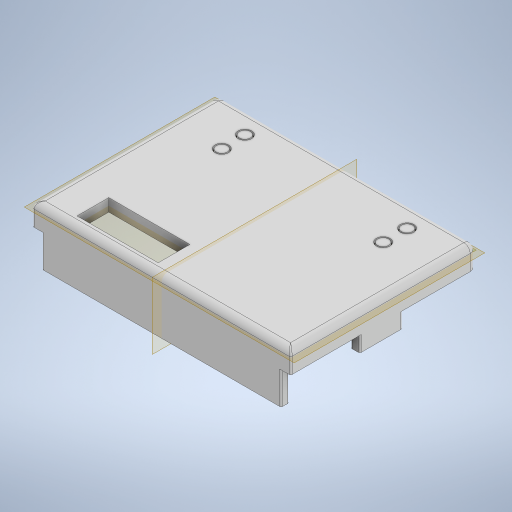
# Autodesk Inventor part: dach
Saved by Autodesk Inventor 2023 (Build 270158000, 158)
## iProperties
Created: 2024-04-28
Part Number: dach
Material: Ogólny
Document SubType Name: Modeling
Designer: kamil
Density: 1 g/cm^3
Appearance: Domyślna
Author: kamil
Autodesk Inventor part; units mm, degrees
ref_plane "YZ Plane" through (0, 0, 0) normal (1, 0, 0) x (0, 1, 0)
ref_plane "XZ Plane" through (0, 0, 0) normal (0, 1, 0) x (-1, 0, 0)
ref_plane "XY Plane" through (0, 0, 0) normal (0, 0, 1) x (1, 0, 0)
sketch "Szkic1" plane through (0, 0, 0) normal (0, 1, 0) x (-1, 0, 0)
  line L0 (41, 29.5365) -> (-41, 29.5365)
  line L1 (-41, 29.5365) -> (-41, -29.5365)
  line L2 (-41, -29.5365) -> (41, -29.5365)
  line L3 (41, -29.5365) -> (41, 29.5365)
  point P0 (0, 0)
  point P1 (41, 0)
  point P2 (0, -29.5365)
  dimension "d0" = 82
  dimension "d1" = 59.073
  constraints: 8 end point, 2 midpoint, 2 parallel, 1 horizontal, 1 horizontal alignment, 1 perpendicular, 1 vertical alignment
  measures "d0" distance of L1.end L2.end
  measures "d1" distance of L2.end L0.start
extrude "Wyciągnięcie proste1" add sketch "Szkic1" along normal blind 4
fillet "Zaokrąglenie2" radius 2 2 edges at (41, 2, -29.5365) (-41, 2, -29.5365)
sketch "Szkic3" plane through (0, 0, 0) normal (0, -1, 0) x (1, 0, 0)
  line L0 (41, 29.5365) -> (41, -29.5365) projected
  line L1 (-41, 29.5365) -> (41, 29.5365) projected
  line L2 (-41, -29.5365) -> (-41, 29.5365) projected
  line L3 (38, 27.0365) -> (-38, 27.0365)
  line L4 (-38, 27.0365) -> (-38, 29.5365)
  line L5 (-38, 29.5365) -> (38, 29.5365)
  line L6 (38, 29.5365) -> (38, 27.0365)
  point P0 (0, 0)
  point P1 (41, 15.9365)
  point P2 (-41, 15.9365)
  point P3 (0, 27.0365)
  point P4 (0, 29.5365)
  point P5 (0, 29.5365)
  point P6 (0, 29.5365)
  dimension "d24" = 76
  dimension "d25" = 2.5
  constraints: 8 end point, 4 midpoint, 2 parallel, 1 coincident, 1 horizontal, 1 perpendicular, 1 vertical alignment
  measures "d24" distance of L4.end L5.end
  measures "d25" distance of L3.end L4.end
extrude "Wyciągnięcie proste3" add sketch "Szkic3" along normal blind 13.3
fillet "Zaokrąglenie5" radius 0.5 2 edges at (-41, 2, 29.5365) (41, 2, 29.5365)
fillet "Zaokrąglenie7" radius 2 8 edges at (40.4142, 4, -28.9507) (0, 4, -29.5365) (-40.4142, 4, -28.9507) (-41, 4, 0.75) (-40.8536, 4, 29.3901) (0, 4, 29.5365) (40.8536, 4, 29.3901) (41, 4, 0.75)
ref_plane "Płaszczyzna konstrukcyjna1" through (0, 1.75, 0) normal (0, 1, 0) x (1, 0, 0)
sketch "Szkic6" plane through (0, 0, 0) normal (0, -1, 0) x (1, 0, 0)
  arc A0 (41, 29.0365) -> (40.5, 29.5365) centre (40.5, 29.0365) ccw projected
  line L0 (38, 29.5365) -> (40.5, 29.5365) projected
  line L1 (38, 29.5365) -> (38, 27.0365) projected
  line L2 (38, 27.0365) -> (-38, 27.0365) projected
  line L3 (-38, 27.0365) -> (-38, 29.5365) projected
  line L4 (-40.5, 29.5365) -> (-38, 29.5365) projected
  arc A1 (-40.5, 29.5365) -> (-41, 29.0365) centre (-40.5, 29.0365) ccw projected
  line L5 (-41, -27.5365) -> (-41, 29.0365) projected
  arc A2 (-41, -27.5365) -> (-39, -29.5365) centre (-39, -27.5365) ccw projected
  line L6 (39, -29.5365) -> (-39, -29.5365) projected
  arc A3 (39, -29.5365) -> (41, -27.5365) centre (39, -27.5365) ccw projected
  line L7 (41, 29.0365) -> (41, -27.5365) projected
  line L8 (-38.1, 24.1365) -> (38.1, 24.1365)
  line L9 (38.1, 24.1365) -> (38.1, -26.6365)
  line L10 (38.1, -26.6365) -> (-38.1, -26.6365)
  line L11 (-38.1, -26.6365) -> (-38.1, 24.1365)
  line L12 (-38.1, 24.1365) -> (-38.1, 32.3252)
  line L13 (38.1, 24.1365) -> (38.1, 40.7001)
  line L14 (38.1, 29.5365) -> (-38.1, 29.5365)
  line L15 (-38.1, 29.5365) -> (-38.1, 27.0365)
  line L16 (-38.1, 27.0365) -> (38.1, 27.0365)
  line L17 (38.1, 27.0365) -> (38.1, 29.5365)
  point P0 (0, 0)
  dimension "d71" = 2.9
  constraints: 20 end point, 3 point on line, 2 parallel, 2 vertical, 1 horizontal, 1 perpendicular, 3 other
  measures "d71" distance between parallel lines of L5 L11
extrude "Wyciągnięcie proste4" add sketch "Szkic6" along normal blind 3 contours L7 A3 L6 A2 L5 A1 L4 L12 L11 L10 L9 L13 L0 A0 | L13 L16 L1 L0 | L1 L2 L3 L14 | L3 L16 L12 L4
sketch "Szkic7" plane through (0, 0, 0) normal (0, -1, 0) x (1, 0, 0)
  circle A0 centre (36.5, 0.75) radius 2 projected
  arc A1 (32, -1.25) -> (36.3571, -6.2085) centre (37, -1.25) ccw projected
  line L0 (32, -1.25) -> (32, 2.75) projected
  arc A2 (36.3571, 7.7085) -> (32, 2.75) centre (37, 2.75) ccw projected
  arc A3 (36.3571, 7.7085) -> (38.1, 9.6919) centre (36.1, 9.6919) ccw projected
  line L1 (38.1, 8.25) -> (38.1, 9.6919) projected
  arc A4 (38.1, 8.25) -> (38.6, 7.75) centre (38.6, 8.25) ccw projected
  line L2 (38.6, 7.75) -> (40.5, 7.75) projected
  arc A5 (40.5, 7.75) -> (41, 8.25) centre (40.5, 8.25) ccw projected
  line L3 (41, 8.25) -> (41, -6.75) projected
  arc A6 (41, -6.75) -> (40.5, -6.25) centre (40.5, -6.75) ccw projected
  line L4 (40.5, -6.25) -> (38.6, -6.25) projected
  arc A7 (38.6, -6.25) -> (38.1, -6.75) centre (38.6, -6.75) ccw projected
  line L5 (38.1, -8.1919) -> (38.1, -6.75) projected
  arc A8 (38.1, -8.1919) -> (36.3571, -6.2085) centre (36.1, -8.1919) ccw projected
  circle A9 centre (36.5, 0.75) radius 1.6 projected
  point P0 (0, 0)
extrude "Wyciągnięcie proste5" add sketch "Szkic7" along normal up to surface (3 mm away) contours A0 | L0 A2 A3 L1 A4 L2 A5 L3 A6 L4 A7 L5 A8 A1
sketch "Szkic8" plane through (0, -3, 0) normal (0, -1, 0) x (1, 0, 0)
  line L0 (38.6, -6.25) -> (40.5, -6.25) projected
  line L1 (40.5, 7.75) -> (38.6, 7.75) projected
  circle A0 centre (36.5, 0.75) radius 2 projected
  arc A1 (32, -1.25) -> (36.3571, -6.2085) centre (37, -1.25) ccw projected
  line L2 (32, -1.25) -> (32, 2.75) projected
  arc A2 (36.3571, 7.7085) -> (32, 2.75) centre (37, 2.75) ccw projected
  arc A3 (36.3571, 7.7085) -> (38.1, 9.6919) centre (36.1, 9.6919) ccw projected
  line L3 (38.1, 8.25) -> (38.1, 9.6919) projected
  arc A4 (38.1, 8.25) -> (38.6, 7.75) centre (38.6, 8.25) ccw projected
  line L4 (38.6, 7.75) -> (40.5, 7.75) projected
  arc A5 (40.5, 7.75) -> (41, 8.25) centre (40.5, 8.25) ccw projected
  line L5 (41, 8.25) -> (41, -6.75) projected
  arc A6 (41, -6.75) -> (40.5, -6.25) centre (40.5, -6.75) ccw projected
  line L6 (40.5, -6.25) -> (38.6, -6.25) projected
  arc A7 (38.6, -6.25) -> (38.1, -6.75) centre (38.6, -6.75) ccw projected
  line L7 (38.1, -8.1919) -> (38.1, -6.75) projected
  arc A8 (38.1, -8.1919) -> (36.3571, -6.2085) centre (36.1, -8.1919) ccw projected
  line L8 (41, -6.05) -> (38.1, -6.05)
  line L9 (38.1, -6.05) -> (38.1, 7.55)
  line L10 (38.1, 7.55) -> (41, 7.55)
  line L11 (41, 7.55) -> (41, -6.05)
  point P0 (0, 0)
  point P1 (41, 0.75)
  point P2 (38.1, 0.75)
  dimension "d76" = 0.2
  dimension "d77" = 0.2
  constraints: 8 end point, 2 midpoint, 2 parallel, 2 vertical alignment, 1 horizontal, 1 perpendicular
  measures "d76" distance between parallel lines of L0 L8
  measures "d77" distance between parallel lines of L1 L10
extrude "Wyciągnięcie proste6" add sketch "Szkic8" along normal blind 4.9 contours L8 L9 A0 L10 L5 | L9 A0 picked at (38.2333, 0.75)
fillet "Zaokrąglenie12" radius 0.5 4 edges at (41, -5.45, 7.55) (38.1, -5.45, 7.55) (41, -5.45, -6.05) (38.1, -5.45, -6.05)
ref_plane "Płaszczyzna konstrukcyjna2" through (0, 2, 29.0365) normal (1, 0, 0) x (0, 0, -1)
mirror "Odbij1" about plane through (0, 2, 29.0365) normal (1, 0, 0) of "Zaokrąglenie12", "Wyciągnięcie proste6", "Wyciągnięcie proste5"
fillet "Zaokrąglenie13" radius 0.5 4 edges at (38, -8.15, 29.5365) (38, -8.15, 27.0365) (-38, -8.15, 27.0365) (-38, -8.15, 29.5365)
fillet "Zaokrąglenie14" radius 1 4 edges at (-38.1, -1.5, 27.0365) (38.1, -1.5, 27.0365) (38.1, -1.5, -26.6365) (-38.1, -1.5, -26.6365)
sketch "Szkic9" plane through (0, 4, 0) normal (0, 1, 0) x (1, 0, 0)
  circle A0 centre (-25.3, 14.8865) radius 1.65 projected
  circle A1 centre (-25.5, 22.4365) radius 1.65 projected
  circle A2 centre (26.05, 14.8365) radius 1.65 projected
  circle A3 centre (26.05, 22.4365) radius 1.65 projected
  line L0 (-28.825, -17.5035) -> (-28.825, -25.6035) projected
  line L1 (-28.825, -25.6035) -> (-8.525, -25.6035) projected
  line L2 (-28.825, -17.5035) -> (-8.525, -17.5035)
  line L3 (-8.525, -17.5035) -> (-8.525, -25.6035)
  line L4 (-8.525, -25.6035) -> (-28.825, -25.6035)
  line L5 (-28.825, -25.6035) -> (-28.825, -17.5035)
  point P0 (0, 0)
  constraints: 8 end point, 2 parallel, 1 horizontal, 1 perpendicular
extrude "Wyciągnięcie proste7" cut sketch "Szkic9" against normal blind 5
sketch "Szkic10" plane through (0, 0, 0) normal (0, -1, 0) x (1, 0, 0)
  circle A0 centre (-25.3, -14.8865) radius 1.65 projected
  circle A1 centre (-25.5, -22.4365) radius 1.65 projected
  circle A2 centre (26.05, -22.4365) radius 1.65 projected
  circle A3 centre (26.05, -14.8365) radius 1.65 projected
  circle A4 centre (-25.5, -22.4365) radius 2.15
  circle A5 centre (-25.3, -14.8865) radius 2.15
  circle A6 centre (26.05, -22.4365) radius 2.15
  circle A7 centre (26.05, -14.8365) radius 2.15
  point P0 (0, 0)
  dimension "d86" = 0.5
  dimension "d87" = 0.5
  dimension "d88" = 0.5
  dimension "d89" = 0.5
  constraints: 4 centre point
  measures "d86" radial gap between concentric circles of A1 A4
  measures "d87" radial gap between concentric circles of A0 A5
  measures "d88" radial gap between concentric circles of A2 A6
  measures "d89" radial gap between concentric circles of A3 A7
extrude "Wyciągnięcie proste8" cut sketch "Szkic10" against normal through all contours A0 | A1 | A2 | A3 | A4 | A5 | A6 | A7
sketch "Szkic11" plane through (0, 4, 0) normal (0, 1, 0) x (1, 0, 0)
  circle A0 centre (-25.5, 22.4365) radius 2.15 projected
  circle A1 centre (-25.3, 14.8865) radius 2.15 projected
  circle A2 centre (26.05, 22.4365) radius 2.15 projected
  circle A3 centre (26.05, 14.8365) radius 2.15 projected
  circle A4 centre (-25.5, 22.4365) radius 1.75
  circle A5 centre (-25.3, 14.8865) radius 1.75
  circle A6 centre (26.05, 22.4365) radius 1.75
  circle A7 centre (26.05, 14.8365) radius 1.75
  point P0 (0, 0)
  dimension "d92" = 3.5
  dimension "d93" = 3.5
  dimension "d94" = 3.5
  dimension "d95" = 3.5
  constraints: 4 centre point, 4 coincident
  measures "d92" diameter of A4
  measures "d93" diameter of A5
  measures "d94" diameter of A6
  measures "d95" diameter of A7
extrude "Wyciągnięcie proste9" add sketch "Szkic11" against normal blind 5 contours A4 | A5 | A6 | A7
ref_plane "Płaszczyzna konstrukcyjna3" through (26.05, -2, -22.4365) normal (0, -1, 0) x (1, 0, 0)
sketch "Szkic14" plane through (0, 0, 0) normal (0, -1, 0) x (1, 0, 0)
  circle A0 centre (26.05, -22.4365) radius 2.15 projected
  circle A1 centre (-25.3, -14.8865) radius 2.15 projected
  circle A2 centre (26.05, -14.8365) radius 2.15 projected
  circle A3 centre (-25.5, -22.4365) radius 2.15 projected
  line L0 (-28.825, 17.5035) -> (-28.825, 25.6035) projected
  line L1 (-28.825, 25.6035) -> (-8.525, 25.6035) projected
  line L2 (-8.525, 25.6035) -> (-8.525, 17.5035) projected
  line L3 (-8.525, 17.5035) -> (-28.825, 17.5035) projected
  circle A4 centre (26.05, -22.4365) radius 3.2
  circle A5 centre (26.05, -14.8365) radius 3.2
  circle A6 centre (-25.5, -22.4365) radius 1.75 projected
  circle A7 centre (-25.5, -22.4365) radius 3.2
  circle A8 centre (-25.3, -14.8865) radius 1.75 projected
  circle A9 centre (-25.3, -14.8865) radius 3.2
  point P0 (0, 0)
  dimension "d108" = 6.4
  dimension "d109" = 6.4
  dimension "d110" = 6.4
  dimension "d111" = 6.4
  constraints: 4 centre point, 4 coincident
  measures "d108" diameter of A4
  measures "d109" diameter of A5
  measures "d110" diameter of A7
  measures "d111" diameter of A9
extrude "Wyciągnięcie proste11" cut sketch "Szkic14" against normal blind 3 contours A4 | A5 | A7 | A9
sketch "Szkic15" plane through (0, 0, 0) normal (0, -1, 0) x (1, 0, 0)
  circle A0 centre (26.05, -22.4365) radius 3.2 projected
  circle A1 centre (26.05, -14.8365) radius 3.2 projected
  circle A2 centre (-25.5, -22.4365) radius 3.2 projected
  circle A3 centre (-25.3, -14.8865) radius 3.2 projected
  line L0 (26.05, -22.4365) -> (26.05, -14.8365) construction
  line L1 (30.25, -22.4365) -> (30.25, -14.8365)
  line L2 (21.85, -14.8365) -> (21.85, -22.4365)
  arc A4 (21.85, -22.4365) -> (30.25, -22.4365) centre (26.05, -22.4365) ccw
  arc A5 (30.25, -14.8365) -> (21.85, -14.8365) centre (26.05, -14.8365) ccw
  line L3 (-37.1, -26.6365) -> (37.1, -26.6365) projected
  circle A6 centre (-25.5, -22.4365) radius 1.75 projected
  line L4 (-25.5, -22.4365) -> (-25.3, -14.8865) construction
  line L5 (-21.2967, -22.5478) -> (-21.0967, -14.9978)
  line L6 (-29.5033, -14.7752) -> (-29.7033, -22.3252)
  arc A7 (-29.7033, -22.3252) -> (-21.2967, -22.5478) centre (-25.5, -22.4365) ccw
  arc A8 (-21.0967, -14.9978) -> (-29.5033, -14.7752) centre (-25.3, -14.8865) ccw
  point P0 (0, 0)
  point P1 (26.05, -18.6365)
  point P2 (-25.4, -18.6615)
  point P3 (-25.7, -26.6365)
  point P4 (-25.3, -26.6365)
  constraints: 16 end point, 9 tangent, 8 point on circle, 4 centre point, 2 midpoint, 2 parallel, 1 vertical, 1 other
extrude "Wyciągnięcie proste12" add sketch "Szkic15" along normal blind 2.5 contours A4 L2 A5 L1 | A7 L6 A8 L5 L3
sketch "Szkic16" plane through (26.05, -1, -22.4365) normal (0, -1, 0) x (1, 0, 0)
  circle A0 centre (0, 0) radius 1.75 projected
  circle A1 centre (0, 7.6) radius 1.75 projected
  circle A2 centre (-51.55, 0) radius 1.75 projected
  circle A3 centre (-51.35, 7.55) radius 1.75 projected
  circle A4 centre (0, 0) radius 2.75
  circle A5 centre (0, 7.6) radius 2.75
  circle A6 centre (-51.55, 0) radius 2.15 projected
  circle A7 centre (-51.55, 0) radius 2.75
  circle A8 centre (-51.35, 7.55) radius 2.75
  point P0 (-26.05, 22.4365)
  dimension "d116" = 5.5
  dimension "d117" = 5.5
  dimension "d118" = 5.5
  dimension "d119" = 5.5
  constraints: 4 centre point, 4 coincident
  measures "d116" diameter of A4
  measures "d117" diameter of A5
  measures "d118" diameter of A7
  measures "d119" diameter of A8
extrude "Wyciągnięcie proste13" add sketch "Szkic16" against normal blind 1 contours A0 | A1 | A2 | A3 | A4 | A5 | A6 | A7 | A8
sketch "Szkic17" plane through (0, -2.5, 0) normal (0, -1, 0) x (1, 0, 0)
  circle A0 centre (26.05, -22.4365) radius 3.2 projected
  circle A1 centre (26.05, -14.8365) radius 3.2 projected
  circle A2 centre (-25.5, -22.4365) radius 3.2 projected
  circle A3 centre (-25.3, -14.8865) radius 3.2 projected
  circle A4 centre (26.05, -14.8365) radius 2.15
  circle A5 centre (26.05, -22.4365) radius 1.75 projected
  circle A6 centre (26.05, -22.4365) radius 2.15
  circle A7 centre (-25.3, -14.8865) radius 2.15
  circle A8 centre (-25.5, -22.4365) radius 2.15
  point P0 (0, 0)
  dimension "d122" = 4.3
  dimension "d123" = 4.3
  dimension "d124" = 4.3
  dimension "d125" = 4.3
  constraints: 4 centre point, 4 coincident
  measures "d122" diameter of A4
  measures "d123" diameter of A6
  measures "d124" diameter of A7
  measures "d125" diameter of A8
extrude "Wyciągnięcie proste14" add sketch "Szkic17" against normal blind 1 contours A0 | A1 | A2 | A3
sketch "Szkic18" plane through (-25.3, -1, -14.8865) normal (0, -1, 0) x (1, 0, 0)
  circle A0 centre (0, 0) radius 2.15 projected
  circle A1 centre (-0.2, -7.55) radius 2.15 projected
  circle A2 centre (51.35, 0.05) radius 2.15 projected
  circle A3 centre (51.35, -7.55) radius 2.15 projected
  circle A4 centre (0, 0) radius 1.75
  circle A5 centre (-0.2, -7.55) radius 1.75
  circle A6 centre (51.35, 0.05) radius 1.75
  circle A7 centre (51.35, -7.55) radius 1.75
  point P0 (25.3, 14.8865)
  dimension "d128" = 3.5
  dimension "d129" = 3.5
  dimension "d130" = 3.5
  dimension "d131" = 3.5
  constraints: 4 centre point, 4 coincident
  measures "d128" diameter of A4
  measures "d129" diameter of A5
  measures "d130" diameter of A6
  measures "d131" diameter of A7
extrude "Wyciągnięcie proste15" add sketch "Szkic18" along normal blind 9.35 contours A4 | A5 | A6 | A7
sketch "Szkic19" plane through (0, 0, 0) normal (0, -1, 0) x (1, 0, 0)
  line L0 (-28.825, 17.5035) -> (-28.825, 25.6035) projected
  line L1 (-28.825, 25.6035) -> (-8.525, 25.6035) projected
  line L2 (-8.525, 25.6035) -> (-8.525, 17.5035) projected
  line L3 (-8.525, 17.5035) -> (-28.825, 17.5035) projected
  arc A0 (-25.3, -26.6365) -> (-21.2967, -22.5478) centre (-25.5, -22.4365) ccw projected
  line L4 (-25.3, -26.6365) -> (26.05, -26.6365) projected
  arc A1 (21.85, -22.4365) -> (26.05, -26.6365) centre (26.05, -22.4365) ccw projected
  line L5 (21.85, -22.4365) -> (21.85, -14.8365) projected
  arc A2 (30.25, -14.8365) -> (21.85, -14.8365) centre (26.05, -14.8365) ccw projected
  line L6 (30.25, -14.8365) -> (30.25, -22.4365) projected
  arc A3 (26.05, -26.6365) -> (30.25, -22.4365) centre (26.05, -22.4365) ccw projected
  line L7 (26.05, -26.6365) -> (37.1, -26.6365) projected
  arc A4 (37.1, -26.6365) -> (38.1, -25.6365) centre (37.1, -25.6365) ccw projected
  line L8 (38.1, -25.6365) -> (38.1, -8.1919) projected
  arc A5 (38.1, -8.1919) -> (36.3571, -6.2085) centre (36.1, -8.1919) ccw projected
  arc A6 (32, -1.25) -> (36.3571, -6.2085) centre (37, -1.25) ccw projected
  line L9 (32, -1.25) -> (32, 2.75) projected
  arc A7 (36.3571, 7.7085) -> (32, 2.75) centre (37, 2.75) ccw projected
  arc A8 (36.3571, 7.7085) -> (38.1, 9.6919) centre (36.1, 9.6919) ccw projected
  line L10 (38.1, 9.6919) -> (38.1, 26.0365) projected
  arc A9 (38.1, 26.0365) -> (37.1, 27.0365) centre (37.1, 26.0365) ccw projected
  line L11 (37.1, 27.0365) -> (-37.1, 27.0365) projected
  arc A10 (-37.1, 27.0365) -> (-38.1, 26.0365) centre (-37.1, 26.0365) ccw projected
  line L12 (-38.1, 26.0365) -> (-38.1, 9.6919) projected
  arc A11 (-38.1, 9.6919) -> (-36.3571, 7.7085) centre (-36.1, 9.6919) ccw projected
  arc A12 (-32, 2.75) -> (-36.3571, 7.7085) centre (-37, 2.75) ccw projected
  line L13 (-32, 2.75) -> (-32, -1.25) projected
  arc A13 (-36.3571, -6.2085) -> (-32, -1.25) centre (-37, -1.25) ccw projected
  arc A14 (-36.3571, -6.2085) -> (-38.1, -8.1919) centre (-36.1, -8.1919) ccw projected
  line L14 (-38.1, -8.1919) -> (-38.1, -25.6365) projected
  arc A15 (-38.1, -25.6365) -> (-37.1, -26.6365) centre (-37.1, -25.6365) ccw projected
  line L15 (-37.1, -26.6365) -> (-25.7, -26.6365) projected
  arc A16 (-29.7033, -22.3252) -> (-25.7, -26.6365) centre (-25.5, -22.4365) ccw projected
  line L16 (-29.7033, -22.3252) -> (-29.5033, -14.7752) projected
  arc A17 (-21.0967, -14.9978) -> (-29.5033, -14.7752) centre (-25.3, -14.8865) ccw projected
  line L17 (-21.0967, -14.9978) -> (-21.2967, -22.5478) projected
  arc A18 (26.05, -26.6365) -> (30.25, -22.4365) centre (26.05, -22.4365) ccw projected
  line L18 (30.25, -22.4365) -> (21.85, -22.4365)
  line L19 (21.85, -22.4365) -> (21.85, -26.6365)
  line L20 (21.85, -26.6365) -> (30.25, -26.6365)
  line L21 (30.25, -26.6365) -> (30.25, -22.4365)
  line L22 (-29.7033, -22.3252) -> (-29.7033, -26.6365)
  line L23 (-21.2967, -22.5478) -> (-21.2967, -26.6365)
  point P0 (0, 0)
  point P1 (21.85, -24.5365)
  point P2 (21.85, -22.4365)
  point P3 (-29.7033, -22.5478)
  constraints: 12 end point, 3 perpendicular, 3 point on line, 2 parallel, 1 horizontal, 1 midpoint, 1 vertical alignment
extrude "Wyciągnięcie proste16" add sketch "Szkic19" along normal up to surface (2.5 mm away) contours A16 L15 L22 | A0 L23 L4 | L19 A1 L4 | A3 L21 L7
sketch "Szkic21" plane through (0, 0, 0) normal (0, -1, 0) x (1, 0, 0)
  line L0 (-28.825, 17.5035) -> (-28.825, 25.6035) projected
  line L1 (-28.825, 25.6035) -> (-8.525, 25.6035) projected
  line L2 (-8.525, 17.5035) -> (-28.825, 17.5035) projected
  line L3 (-8.525, 25.6035) -> (-8.525, 17.5035) projected
  line L4 (-8.525, 25.6035) -> (-5.025, 25.6035)
  line L5 (-5.025, 25.6035) -> (-5.025, 17.5035)
  line L6 (-5.025, 17.5035) -> (-8.525, 17.5035)
  line L7 (-8.525, 17.5035) -> (-8.525, 25.6035)
  line L8 (-29.825, 16.5035) -> (-29.825, 26.6035)
  line L9 (-29.825, 26.6035) -> (-7.525, 26.6035)
  line L10 (-7.525, 26.6035) -> (-7.525, 16.5035)
  line L11 (-7.525, 16.5035) -> (-29.825, 16.5035)
  line L12 (-9.525, 16.5035) -> (-4.025, 16.5035)
  line L13 (-4.025, 16.5035) -> (-4.025, 26.6035)
  line L14 (-4.025, 26.6035) -> (-9.525, 26.6035)
  line L15 (-9.525, 26.6035) -> (-9.525, 16.5035)
  point P0 (0, 0)
  point P1 (-6.775, 17.5035)
  point P2 (-7.525, 26.6035)
  dimension "d140" = 3.5
  dimension "d141" = 1
  dimension "d142" = 1
  constraints: 24 end point, 4 parallel, 2 perpendicular, 1 horizontal, 1 horizontal alignment, 1 midpoint, 6 other
  measures "d140" distance between parallel lines of L5 L3
  measures "d141" distance between parallel lines of L2 L11
  measures "d142" distance between parallel lines of L6 L12
extrude "Wyciągnięcie proste18" cut sketch "Szkic21" against normal blind 10
